Autodesk Fusion 360 part; units mm, degrees
(part 5 of 8)
  line L594 (-322.3503, 58.85) -> (-319.3503, 58.85)
  line L595 (-319.3503, 58.85) -> (-319.3503, 55.85)
  line L596 (-319.3503, 55.85) -> (-322.3503, 55.85)
  line L597 (-322.3503, 55.85) -> (-322.3503, 52.85)
  line L598 (-322.3503, 52.85) -> (-319.3503, 52.85)
  line L599 (-319.3503, 52.85) -> (-319.3503, 49.85)
  line L600 (-319.3503, 49.85) -> (-322.3503, 49.85)
  line L601 (-322.3503, 49.85) -> (-322.3503, 46.85)
  line L602 (-322.3503, 46.85) -> (-319.3503, 46.85)
  line L603 (-319.3503, 46.85) -> (-319.3503, 43.85)
  line L604 (-319.3503, 43.85) -> (-322.3503, 43.85)
  line L605 (-322.3503, 43.85) -> (-322.3503, 40.85)
  line L606 (-322.3503, 40.85) -> (-319.3503, 40.85)
  line L607 (-319.3503, 40.85) -> (-319.3503, 37.85)
  line L608 (-319.3503, 37.85) -> (-322.3503, 37.85)
  line L609 (-322.3503, 37.85) -> (-322.3503, 34.85)
  line L610 (-322.3503, 34.85) -> (-319.3503, 34.85)
  line L611 (-319.3503, 34.85) -> (-319.3503, 31.85)
  circle A0 centre (-110.4882, 52.6046) radius 2.5
  circle A1 centre (-197.9882, 140.1046) radius 2.5
  circle A2 centre (-210.4882, 152.6046) radius 2.5
  circle A3 centre (-122.9882, 65.1046) radius 2.5
  circle A4 centre (-122.9882, 140.1046) radius 2.5
  circle A5 centre (-197.9882, 65.1046) radius 2.5
  circle A6 centre (-210.4882, 52.6046) radius 2.5
  circle A7 centre (-110.4882, 152.6046) radius 2.5
sketch "Sketch8" plane through (0, 3, 0) normal (0, 1, 0) x (-1, 0, 0)
  line L0 (-319.3503, 31.85) -> (-322.3503, 31.85)
  line L1 (-322.3503, 31.85) -> (-322.3503, 28.1)
  line L2 (-322.3503, 28.1) -> (-319.3503, 28.1)
  line L3 (-319.3503, 28.1) -> (-319.3503, 27.35)
  line L4 (-319.3503, 27.35) -> (-317.6003, 27.35)
  line L5 (-317.6003, 27.35) -> (-317.6003, 24.35)
  line L6 (-317.6003, 24.35) -> (-312.8503, 24.35)
  line L7 (-312.8503, 24.35) -> (-312.8503, 27.35)
  line L8 (-312.8503, 27.35) -> (-309.8503, 27.35)
  line L9 (-309.8503, 27.35) -> (-309.8503, 24.35)
  line L10 (-309.8503, 24.35) -> (-306.8503, 24.35)
  line L11 (-306.8503, 24.35) -> (-306.8503, 27.35)
  line L12 (-306.8503, 27.35) -> (-303.8502, 27.35)
  line L13 (-303.8502, 27.35) -> (-303.8502, 24.35)
  line L14 (-303.8502, 24.35) -> (-300.8502, 24.35)
  line L15 (-300.8502, 24.35) -> (-300.8502, 27.35)
  line L16 (-300.8502, 27.35) -> (-297.8502, 27.35)
  line L17 (-297.8502, 27.35) -> (-297.8502, 24.35)
  line L18 (-297.8502, 24.35) -> (-294.8502, 24.35)
  line L19 (-294.8502, 24.35) -> (-294.8502, 27.35)
  line L20 (-294.8502, 27.35) -> (-291.8502, 27.35)
  line L21 (-291.8502, 27.35) -> (-291.8502, 24.35)
  line L22 (-291.8502, 24.35) -> (-288.8502, 24.35)
  line L23 (-288.8502, 24.35) -> (-288.8502, 27.35)
  line L24 (-288.8502, 27.35) -> (-285.8502, 27.35)
  line L25 (-285.8502, 27.35) -> (-285.8502, 24.35)
  line L26 (-285.8502, 24.35) -> (-282.8502, 24.35)
  line L27 (-282.8502, 24.35) -> (-282.8502, 27.35)
  line L28 (-282.8502, 27.35) -> (-279.8502, 27.35)
  line L29 (-279.8502, 27.35) -> (-279.8502, 24.35)
  line L30 (-279.8502, 24.35) -> (-276.8502, 24.35)
  line L31 (-276.8502, 24.35) -> (-276.8502, 27.35)
  line L32 (-276.8502, 27.35) -> (-273.8502, 27.35)
  line L33 (-273.8502, 27.35) -> (-273.8502, 24.35)
  line L34 (-273.8502, 24.35) -> (-270.8502, 24.35)
  line L35 (-270.8502, 24.35) -> (-270.8502, 27.35)
  line L36 (-270.8502, 27.35) -> (-267.8502, 27.35)
  line L37 (-267.8502, 27.35) -> (-267.8502, 24.35)
  line L38 (-267.8502, 24.35) -> (-264.8502, 24.35)
  line L39 (-264.8502, 24.35) -> (-264.8502, 27.35)
  line L40 (-264.8502, 27.35) -> (-261.8502, 27.35)
  line L41 (-261.8502, 27.35) -> (-261.8502, 24.35)
  line L42 (-261.8502, 24.35) -> (-258.8502, 24.35)
  line L43 (-258.8502, 24.35) -> (-258.8502, 27.35)
  line L44 (-258.8502, 27.35) -> (-255.8502, 27.35)
  line L45 (-255.8502, 27.35) -> (-255.8502, 24.35)
  line L46 (-255.8502, 24.35) -> (-252.8502, 24.35)
  line L47 (-252.8502, 24.35) -> (-252.8502, 27.35)
  line L48 (-252.8502, 27.35) -> (-249.8502, 27.35)
  line L49 (-249.8502, 27.35) -> (-249.8502, 24.35)
  line L50 (-249.8502, 24.35) -> (-246.8502, 24.35)
  line L51 (-246.8502, 24.35) -> (-246.8502, 27.35)
  line L52 (-246.8502, 27.35) -> (-243.8502, 27.35)
  line L53 (-243.8502, 27.35) -> (-243.8502, 24.35)
  line L54 (-243.8502, 24.35) -> (-240.8502, 24.35)
  line L55 (-240.8502, 24.35) -> (-240.8502, 27.35)
  line L56 (-240.8502, 27.35) -> (-237.8502, 27.35)
  line L57 (-237.8502, 27.35) -> (-237.8502, 24.35)
  line L58 (-237.8502, 24.35) -> (-234.8502, 24.35)
  line L59 (-234.8502, 24.35) -> (-234.8502, 27.35)
  line L60 (-234.8502, 27.35) -> (-231.8502, 27.35)
  line L61 (-231.8502, 27.35) -> (-231.8502, 24.35)
  line L62 (-231.8502, 24.35) -> (-228.8502, 24.35)
  line L63 (-228.8502, 24.35) -> (-228.8502, 27.35)
  line L64 (-228.8502, 27.35) -> (-225.8502, 27.35)
  line L65 (-225.8502, 27.35) -> (-225.8502, 24.35)
  line L66 (-225.8502, 24.35) -> (-222.8502, 24.35)
  line L67 (-222.8502, 24.35) -> (-222.8502, 27.35)
  line L68 (-222.8502, 27.35) -> (-219.8502, 27.35)
  line L69 (-219.8502, 27.35) -> (-219.8502, 24.35)
  line L70 (-219.8502, 24.35) -> (-216.8502, 24.35)
  line L71 (-216.8502, 24.35) -> (-216.8502, 27.35)
  line L72 (-216.8502, 27.35) -> (-213.8502, 27.35)
  line L73 (-213.8502, 27.35) -> (-213.8502, 24.35)
  line L74 (-213.8502, 24.35) -> (-210.8502, 24.35)
  line L75 (-210.8502, 24.35) -> (-210.8502, 27.35)
  line L76 (-210.8502, 27.35) -> (-207.8502, 27.35)
  line L77 (-207.8502, 27.35) -> (-207.8502, 24.35)
  line L78 (-207.8502, 24.35) -> (-204.8502, 24.35)
  line L79 (-204.8502, 24.35) -> (-204.8502, 27.35)
  line L80 (-204.8502, 27.35) -> (-201.8502, 27.35)
  line L81 (-201.8502, 27.35) -> (-201.8502, 24.35)
  line L82 (-201.8502, 24.35) -> (-198.8502, 24.35)
  line L83 (-198.8502, 24.35) -> (-198.8502, 27.35)
  line L84 (-198.8502, 27.35) -> (-195.8502, 27.35)
  line L85 (-195.8502, 27.35) -> (-195.8502, 24.35)
  line L86 (-195.8502, 24.35) -> (-192.8502, 24.35)
  line L87 (-192.8502, 24.35) -> (-192.8502, 27.35)
  line L88 (-192.8502, 27.35) -> (-189.8502, 27.35)
  line L89 (-189.8502, 27.35) -> (-189.8502, 24.35)
  line L90 (-189.8502, 24.35) -> (-186.8502, 24.35)
  line L91 (-186.8502, 24.35) -> (-186.8502, 27.35)
  line L92 (-186.8502, 27.35) -> (-183.8502, 27.35)
  line L93 (-183.8502, 27.35) -> (-183.8502, 24.35)
  line L94 (-183.8502, 24.35) -> (-180.8501, 24.35)
  line L95 (-180.8501, 24.35) -> (-180.8501, 27.35)
  line L96 (-180.8501, 27.35) -> (-177.8501, 27.35)
  line L97 (-177.8501, 27.35) -> (-177.8501, 24.35)
  line L98 (-177.8501, 24.35) -> (-174.8501, 24.35)
  line L99 (-174.8501, 24.35) -> (-174.8501, 27.35)
  line L100 (-174.8501, 27.35) -> (-171.8501, 27.35)
  line L101 (-171.8501, 27.35) -> (-171.8501, 24.35)
  line L102 (-171.8501, 24.35) -> (-168.8501, 24.35)
  line L103 (-168.8501, 24.35) -> (-168.8501, 27.35)
  line L104 (-168.8501, 27.35) -> (-165.8501, 27.35)
  line L105 (-165.8501, 27.35) -> (-165.8501, 24.35)
  line L106 (-165.8501, 24.35) -> (-162.8501, 24.35)
  line L107 (-162.8501, 24.35) -> (-162.8501, 27.35)
  line L108 (-162.8501, 27.35) -> (-159.8501, 27.35)
  line L109 (-159.8501, 27.35) -> (-159.8501, 24.35)
  line L110 (-159.8501, 24.35) -> (-156.8501, 24.35)
  line L111 (-156.8501, 24.35) -> (-156.8501, 27.35)
  line L112 (-156.8501, 27.35) -> (-153.8501, 27.35)
  line L113 (-153.8501, 27.35) -> (-153.8501, 24.35)
  line L114 (-153.8501, 24.35) -> (-150.8501, 24.35)
  line L115 (-150.8501, 24.35) -> (-150.8501, 27.35)
  line L116 (-150.8501, 27.35) -> (-147.8501, 27.35)
  line L117 (-147.8501, 27.35) -> (-147.8501, 24.35)
  line L118 (-147.8501, 24.35) -> (-144.8501, 24.35)
  line L119 (-144.8501, 24.35) -> (-144.8501, 27.35)
  line L120 (-144.8501, 27.35) -> (-141.8501, 27.35)
  line L121 (-141.8501, 27.35) -> (-141.8501, 24.35)
  line L122 (-141.8501, 24.35) -> (-138.8501, 24.35)
  line L123 (-138.8501, 24.35) -> (-138.8501, 27.35)
  line L124 (-138.8501, 27.35) -> (-135.8501, 27.35)
  line L125 (-135.8501, 27.35) -> (-135.8501, 24.35)
  line L126 (-135.8501, 24.35) -> (-132.8501, 24.35)
  line L127 (-132.8501, 24.35) -> (-132.8501, 27.35)
  line L128 (-132.8501, 27.35) -> (-129.8501, 27.35)
  line L129 (-129.8501, 27.35) -> (-129.8501, 24.35)
  line L130 (-129.8501, 24.35) -> (-126.8501, 24.35)
  line L131 (-126.8501, 24.35) -> (-126.8501, 27.35)
  line L132 (-126.8501, 27.35) -> (-123.8501, 27.35)
  line L133 (-123.8501, 27.35) -> (-123.8501, 24.35)
  line L134 (-123.8501, 24.35) -> (-120.8501, 24.35)
  line L135 (-120.8501, 24.35) -> (-120.8501, 27.35)
  line L136 (-120.8501, 27.35) -> (-117.8501, 27.35)
  line L137 (-117.8501, 27.35) -> (-117.8501, 24.35)
  line L138 (-117.8501, 24.35) -> (-114.8501, 24.35)
  line L139 (-114.8501, 24.35) -> (-114.8501, 27.35)
  line L140 (-114.8501, 27.35) -> (-111.8501, 27.35)
  line L141 (-111.8501, 27.35) -> (-111.8501, 24.35)
  line L142 (-111.8501, 24.35) -> (-108.8501, 24.35)
  line L143 (-108.8501, 24.35) -> (-108.8501, 27.35)
  line L144 (-108.8501, 27.35) -> (-105.8501, 27.35)
  line L145 (-105.8501, 27.35) -> (-105.8501, 24.35)
  line L146 (-105.8501, 24.35) -> (-102.8501, 24.35)
  line L147 (-102.8501, 24.35) -> (-102.8501, 27.35)
  line L148 (-102.8501, 27.35) -> (-99.8501, 27.35)
  line L149 (-99.8501, 27.35) -> (-99.8501, 24.35)
  line L150 (-99.8501, 24.35) -> (-96.8501, 24.35)
  line L151 (-96.8501, 24.35) -> (-96.8501, 27.35)
  line L152 (-96.8501, 27.35) -> (-93.8501, 27.35)
  line L153 (-93.8501, 27.35) -> (-93.8501, 24.35)
  line L154 (-93.8501, 24.35) -> (-90.8501, 24.35)
  line L155 (-90.8501, 24.35) -> (-90.8501, 27.35)
  line L156 (-90.8501, 27.35) -> (-87.8501, 27.35)
  line L157 (-87.8501, 27.35) -> (-87.8501, 24.35)
  line L158 (-87.8501, 24.35) -> (-84.8501, 24.35)
  line L159 (-84.8501, 24.35) -> (-84.8501, 27.35)
  line L160 (-84.8501, 27.35) -> (-81.8501, 27.35)
  line L161 (-81.8501, 27.35) -> (-81.8501, 24.35)
  line L162 (-81.8501, 24.35) -> (-78.8501, 24.35)
  line L163 (-78.8501, 24.35) -> (-78.8501, 27.35)
  line L164 (-78.8501, 27.35) -> (-75.8501, 27.35)
  line L165 (-75.8501, 27.35) -> (-75.8501, 24.35)
  line L166 (-75.8501, 24.35) -> (-72.8501, 24.35)
  line L167 (-72.8501, 24.35) -> (-72.8501, 27.35)
  line L168 (-72.8501, 27.35) -> (-69.8501, 27.35)
  line L169 (-69.8501, 27.35) -> (-69.8501, 24.35)
  line L170 (-69.8501, 24.35) -> (-66.8501, 24.35)
  line L171 (-66.8501, 24.35) -> (-66.8501, 27.35)
  line L172 (-66.8501, 27.35) -> (-63.8501, 27.35)
  line L173 (-63.8501, 27.35) -> (-63.8501, 24.35)
  line L174 (-63.8501, 24.35) -> (-60.8501, 24.35)
  line L175 (-60.8501, 24.35) -> (-60.8501, 27.35)
  line L176 (-60.8501, 27.35) -> (-57.85, 27.35)
  line L177 (-57.85, 27.35) -> (-57.85, 24.35)
  line L178 (-57.85, 24.35) -> (-54.85, 24.35)
  line L179 (-54.85, 24.35) -> (-54.85, 27.35)
  line L180 (-54.85, 27.35) -> (-51.85, 27.35)
  line L181 (-51.85, 27.35) -> (-51.85, 24.35)
  line L182 (-51.85, 24.35) -> (-48.85, 24.35)
  line L183 (-48.85, 24.35) -> (-48.85, 27.35)
  line L184 (-48.85, 27.35) -> (-45.85, 27.35)
  line L185 (-45.85, 27.35) -> (-45.85, 24.35)
  line L186 (-45.85, 24.35) -> (-42.85, 24.35)
  line L187 (-42.85, 24.35) -> (-42.85, 27.35)
  line L188 (-42.85, 27.35) -> (-39.85, 27.35)
  line L189 (-39.85, 27.35) -> (-39.85, 24.35)
  line L190 (-39.85, 24.35) -> (-36.85, 24.35)
  line L191 (-36.85, 24.35) -> (-36.85, 27.35)
  line L192 (-36.85, 27.35) -> (-33.85, 27.35)
  line L193 (-33.85, 27.35) -> (-33.85, 24.35)
  line L194 (-33.85, 24.35) -> (-30.85, 24.35)
  line L195 (-30.85, 24.35) -> (-30.85, 27.35)
  line L196 (-30.85, 27.35) -> (-27.85, 27.35)
  line L197 (-27.85, 27.35) -> (-27.85, 24.35)
  line L198 (-27.85, 24.35) -> (-24.85, 24.35)
  line L199 (-24.85, 24.35) -> (-24.85, 27.35)
  line L200 (-24.85, 27.35) -> (-21.85, 27.35)
  line L201 (-21.85, 27.35) -> (-21.85, 24.35)
  line L202 (-21.85, 24.35) -> (-18.85, 24.35)
  line L203 (-18.85, 24.35) -> (-18.85, 27.35)
  line L204 (-18.85, 27.35) -> (-15.85, 27.35)
  line L205 (-15.85, 27.35) -> (-15.85, 24.35)
  line L206 (-15.85, 24.35) -> (-11.1, 24.35)
  line L207 (-11.1, 24.35) -> (-11.1, 27.35)
  line L208 (-11.1, 27.35) -> (-9.35, 27.35)
  line L209 (-9.35, 27.35) -> (-9.35, 28.1)
  line L210 (-9.35, 28.1) -> (-6.35, 28.1)
  line L211 (-6.35, 28.1) -> (-6.35, 31.85)
  line L212 (-6.35, 31.85) -> (-9.35, 31.85)
  line L213 (-9.35, 31.85) -> (-9.35, 34.85)
  line L214 (-9.35, 34.85) -> (-6.35, 34.85)
  line L215 (-6.35, 34.85) -> (-6.35, 37.85)
  line L216 (-6.35, 37.85) -> (-9.35, 37.85)
  line L217 (-9.35, 37.85) -> (-9.35, 40.85)
  line L218 (-9.35, 40.85) -> (-6.35, 40.85)
  line L219 (-6.35, 40.85) -> (-6.35, 43.85)
  line L220 (-6.35, 43.85) -> (-9.35, 43.85)
  line L221 (-9.35, 43.85) -> (-9.35, 46.85)
  line L222 (-9.35, 46.85) -> (-6.35, 46.85)
  line L223 (-6.35, 46.85) -> (-6.35, 49.85)
  line L224 (-6.35, 49.85) -> (-9.35, 49.85)
  line L225 (-9.35, 49.85) -> (-9.35, 52.85)
  line L226 (-9.35, 52.85) -> (-6.35, 52.85)
  line L227 (-6.35, 52.85) -> (-6.35, 55.85)
  line L228 (-6.35, 55.85) -> (-9.35, 55.85)
  line L229 (-9.35, 55.85) -> (-9.35, 58.85)
  line L230 (-9.35, 58.85) -> (-6.35, 58.85)
  line L231 (-6.35, 58.85) -> (-6.35, 61.8501)
  line L232 (-6.35, 61.8501) -> (-9.35, 61.8501)
  line L233 (-9.35, 61.8501) -> (-9.35, 64.8501)
  line L234 (-9.35, 64.8501) -> (-6.35, 64.8501)
  line L235 (-6.35, 64.8501) -> (-6.35, 67.8501)
  line L236 (-6.35, 67.8501) -> (-9.35, 67.8501)
  line L237 (-9.35, 67.8501) -> (-9.35, 70.8501)
  line L238 (-9.35, 70.8501) -> (-6.35, 70.8501)
  line L239 (-6.35, 70.8501) -> (-6.35, 73.8501)
  line L240 (-6.35, 73.8501) -> (-9.35, 73.8501)
  line L241 (-9.35, 73.8501) -> (-9.35, 76.8501)
  line L242 (-9.35, 76.8501) -> (-6.35, 76.8501)
  line L243 (-6.35, 76.8501) -> (-6.35, 79.8501)
  line L244 (-6.35, 79.8501) -> (-9.35, 79.8501)
  line L245 (-9.35, 79.8501) -> (-9.35, 82.8501)
  line L246 (-9.35, 82.8501) -> (-6.35, 82.8501)
  line L247 (-6.35, 82.8501) -> (-6.35, 85.8501)
  line L248 (-6.35, 85.8501) -> (-9.35, 85.8501)
  line L249 (-9.35, 85.8501) -> (-9.35, 88.8501)
  line L250 (-9.35, 88.8501) -> (-6.35, 88.8501)
  line L251 (-6.35, 88.8501) -> (-6.35, 91.8501)
  line L252 (-6.35, 91.8501) -> (-9.35, 91.8501)
  line L253 (-9.35, 91.8501) -> (-9.35, 94.8501)
  line L254 (-9.35, 94.8501) -> (-6.35, 94.8501)
  line L255 (-6.35, 94.8501) -> (-6.35, 97.8501)
  line L256 (-6.35, 97.8501) -> (-9.35, 97.8501)
  line L257 (-9.35, 97.8501) -> (-9.35, 100.8501)
  line L258 (-9.35, 100.8501) -> (-6.35, 100.8501)
  line L259 (-6.35, 100.8501) -> (-6.35, 103.8501)
  line L260 (-6.35, 103.8501) -> (-9.35, 103.8501)
  line L261 (-9.35, 103.8501) -> (-9.35, 106.8501)
  line L262 (-9.35, 106.8501) -> (-6.35, 106.8501)
  line L263 (-6.35, 106.8501) -> (-6.35, 109.8501)
  line L264 (-6.35, 109.8501) -> (-9.35, 109.8501)
  line L265 (-9.35, 109.8501) -> (-9.35, 112.8501)
  line L266 (-9.35, 112.8501) -> (-6.35, 112.8501)
  line L267 (-6.35, 112.8501) -> (-6.35, 115.8501)
  line L268 (-6.35, 115.8501) -> (-9.35, 115.8501)
  line L269 (-9.35, 115.8501) -> (-9.35, 118.8501)
  line L270 (-9.35, 118.8501) -> (-6.35, 118.8501)
  line L271 (-6.35, 118.8501) -> (-6.35, 121.8501)
  line L272 (-6.35, 121.8501) -> (-9.35, 121.8501)
  line L273 (-9.35, 121.8501) -> (-9.35, 124.8501)
  line L274 (-9.35, 124.8501) -> (-6.35, 124.8501)
  line L275 (-6.35, 124.8501) -> (-6.35, 127.8501)
  line L276 (-6.35, 127.8501) -> (-9.35, 127.8501)
  line L277 (-9.35, 127.8501) -> (-9.35, 130.8501)
  line L278 (-9.35, 130.8501) -> (-6.35, 130.8501)
  line L279 (-6.35, 130.8501) -> (-6.35, 133.8501)
  line L280 (-6.35, 133.8501) -> (-9.35, 133.8501)
  line L281 (-9.35, 133.8501) -> (-9.35, 136.8501)
  line L282 (-9.35, 136.8501) -> (-6.35, 136.8501)
  line L283 (-6.35, 136.8501) -> (-6.35, 139.8501)
  line L284 (-6.35, 139.8501) -> (-9.35, 139.8501)
  line L285 (-9.35, 139.8501) -> (-9.35, 142.8501)
  line L286 (-9.35, 142.8501) -> (-6.35, 142.8501)
  line L287 (-6.35, 142.8501) -> (-6.35, 145.8501)
  line L288 (-6.35, 145.8501) -> (-9.35, 145.8501)
  line L289 (-9.35, 145.8501) -> (-9.35, 148.8501)
  line L290 (-9.35, 148.8501) -> (-6.35, 148.8501)
  line L291 (-6.35, 148.8501) -> (-6.35, 151.8501)
  line L292 (-6.35, 151.8501) -> (-9.35, 151.8501)
  line L293 (-9.35, 151.8501) -> (-9.35, 154.8501)
  line L294 (-9.35, 154.8501) -> (-6.35, 154.8501)
  line L295 (-6.35, 154.8501) -> (-6.35, 157.8501)
  line L296 (-6.35, 157.8501) -> (-9.35, 157.8501)
  line L297 (-9.35, 157.8501) -> (-9.35, 160.8501)
  line L298 (-9.35, 160.8501) -> (-6.35, 160.8501)
  line L299 (-6.35, 160.8501) -> (-6.35, 163.8501)
  line L300 (-6.35, 163.8501) -> (-9.35, 163.8501)
  line L301 (-9.35, 163.8501) -> (-9.35, 166.8501)
  line L302 (-9.35, 166.8501) -> (-6.35, 166.8501)
  line L303 (-6.35, 166.8501) -> (-6.35, 169.8501)
  line L304 (-6.35, 169.8501) -> (-9.35, 169.8501)
  line L305 (-9.35, 169.8501) -> (-9.35, 172.8501)
  line L306 (-9.35, 172.8501) -> (-6.35, 172.8501)
  line L307 (-6.35, 172.8501) -> (-6.35, 176.6001)
  line L308 (-6.35, 176.6001) -> (-9.35, 176.6001)
  line L309 (-9.35, 176.6001) -> (-9.35, 177.3501)
  line L310 (-9.35, 177.3501) -> (-11.1, 177.3501)
  line L311 (-11.1, 177.3501) -> (-11.1, 180.3501)
  line L312 (-11.1, 180.3501) -> (-15.85, 180.3501)
  line L313 (-15.85, 180.3501) -> (-15.85, 177.3501)
  line L314 (-15.85, 177.3501) -> (-18.85, 177.3501)
  line L315 (-18.85, 177.3501) -> (-18.85, 180.3501)
  line L316 (-18.85, 180.3501) -> (-21.85, 180.3501)
  line L317 (-21.85, 180.3501) -> (-21.85, 177.3501)
  line L318 (-21.85, 177.3501) -> (-24.85, 177.3501)
  line L319 (-24.85, 177.3501) -> (-24.85, 180.3501)
  line L320 (-24.85, 180.3501) -> (-27.85, 180.3501)
  line L321 (-27.85, 180.3501) -> (-27.85, 177.3501)
  line L322 (-27.85, 177.3501) -> (-30.85, 177.3501)
  line L323 (-30.85, 177.3501) -> (-30.85, 180.3501)
  line L324 (-30.85, 180.3501) -> (-33.85, 180.3501)
  line L325 (-33.85, 180.3501) -> (-33.85, 177.3501)
  line L326 (-33.85, 177.3501) -> (-36.85, 177.3501)
  line L327 (-36.85, 177.3501) -> (-36.85, 180.3501)
  line L328 (-36.85, 180.3501) -> (-39.85, 180.3501)
  line L329 (-39.85, 180.3501) -> (-39.85, 177.3501)
  line L330 (-39.85, 177.3501) -> (-42.85, 177.3501)
  line L331 (-42.85, 177.3501) -> (-42.85, 180.3501)
  line L332 (-42.85, 180.3501) -> (-45.85, 180.3501)
  line L333 (-45.85, 180.3501) -> (-45.85, 177.3501)
  line L334 (-45.85, 177.3501) -> (-48.85, 177.3501)
  line L335 (-48.85, 177.3501) -> (-48.85, 180.3501)
  line L336 (-48.85, 180.3501) -> (-51.85, 180.3501)
  line L337 (-51.85, 180.3501) -> (-51.85, 177.3501)
  line L338 (-51.85, 177.3501) -> (-54.85, 177.3501)
  line L339 (-54.85, 177.3501) -> (-54.85, 180.3501)
  line L340 (-54.85, 180.3501) -> (-57.85, 180.3501)
  line L341 (-57.85, 180.3501) -> (-57.85, 177.3501)
  line L342 (-57.85, 177.3501) -> (-60.8501, 177.3501)
  line L343 (-60.8501, 177.3501) -> (-60.8501, 180.3501)
  line L344 (-60.8501, 180.3501) -> (-63.8501, 180.3501)
  line L345 (-63.8501, 180.3501) -> (-63.8501, 177.3501)
  line L346 (-63.8501, 177.3501) -> (-66.8501, 177.3501)
  line L347 (-66.8501, 177.3501) -> (-66.8501, 180.3501)
  line L348 (-66.8501, 180.3501) -> (-69.8501, 180.3501)
  line L349 (-69.8501, 180.3501) -> (-69.8501, 177.3501)
  line L350 (-69.8501, 177.3501) -> (-72.8501, 177.3501)
  line L351 (-72.8501, 177.3501) -> (-72.8501, 180.3501)
  line L352 (-72.8501, 180.3501) -> (-75.8501, 180.3501)
  line L353 (-75.8501, 180.3501) -> (-75.8501, 177.3501)
  line L354 (-75.8501, 177.3501) -> (-78.8501, 177.3501)
  line L355 (-78.8501, 177.3501) -> (-78.8501, 180.3501)
  line L356 (-78.8501, 180.3501) -> (-81.8501, 180.3501)
  line L357 (-81.8501, 180.3501) -> (-81.8501, 177.3501)
  line L358 (-81.8501, 177.3501) -> (-84.8501, 177.3501)
  line L359 (-84.8501, 177.3501) -> (-84.8501, 180.3501)
  line L360 (-84.8501, 180.3501) -> (-87.8501, 180.3501)
  line L361 (-87.8501, 180.3501) -> (-87.8501, 177.3501)
  line L362 (-87.8501, 177.3501) -> (-90.8501, 177.3501)
  line L363 (-90.8501, 177.3501) -> (-90.8501, 180.3501)
  line L364 (-90.8501, 180.3501) -> (-93.8501, 180.3501)
  line L365 (-93.8501, 180.3501) -> (-93.8501, 177.3501)
  line L366 (-93.8501, 177.3501) -> (-96.8501, 177.3501)
  line L367 (-96.8501, 177.3501) -> (-96.8501, 180.3501)
  line L368 (-96.8501, 180.3501) -> (-99.8501, 180.3501)
  line L369 (-99.8501, 180.3501) -> (-99.8501, 177.3501)
  line L370 (-99.8501, 177.3501) -> (-102.8501, 177.3501)
  line L371 (-102.8501, 177.3501) -> (-102.8501, 180.3501)
  line L372 (-102.8501, 180.3501) -> (-105.8501, 180.3501)
  line L373 (-105.8501, 180.3501) -> (-105.8501, 177.3501)
  line L374 (-105.8501, 177.3501) -> (-108.8501, 177.3501)
  line L375 (-108.8501, 177.3501) -> (-108.8501, 180.3501)
  line L376 (-108.8501, 180.3501) -> (-111.8501, 180.3501)
  line L377 (-111.8501, 180.3501) -> (-111.8501, 177.3501)
  line L378 (-111.8501, 177.3501) -> (-114.8501, 177.3501)
  line L379 (-114.8501, 177.3501) -> (-114.8501, 180.3501)
  line L380 (-114.8501, 180.3501) -> (-117.8501, 180.3501)
  line L381 (-117.8501, 180.3501) -> (-117.8501, 177.3501)
  line L382 (-117.8501, 177.3501) -> (-120.8501, 177.3501)
  line L383 (-120.8501, 177.3501) -> (-120.8501, 180.3501)
  line L384 (-120.8501, 180.3501) -> (-123.8501, 180.3501)
  line L385 (-123.8501, 180.3501) -> (-123.8501, 177.3501)
  line L386 (-123.8501, 177.3501) -> (-126.8501, 177.3501)
  line L387 (-126.8501, 177.3501) -> (-126.8501, 180.3501)
  line L388 (-126.8501, 180.3501) -> (-129.8501, 180.3501)
  line L389 (-129.8501, 180.3501) -> (-129.8501, 177.3501)
  line L390 (-129.8501, 177.3501) -> (-132.8501, 177.3501)
  line L391 (-132.8501, 177.3501) -> (-132.8501, 180.3501)
  line L392 (-132.8501, 180.3501) -> (-135.8501, 180.3501)
  line L393 (-135.8501, 180.3501) -> (-135.8501, 177.3501)
  line L394 (-135.8501, 177.3501) -> (-138.8501, 177.3501)
  line L395 (-138.8501, 177.3501) -> (-138.8501, 180.3501)
  line L396 (-138.8501, 180.3501) -> (-141.8501, 180.3501)
  line L397 (-141.8501, 180.3501) -> (-141.8501, 177.3501)
  line L398 (-141.8501, 177.3501) -> (-144.8501, 177.3501)
  line L399 (-144.8501, 177.3501) -> (-144.8501, 180.3501)
  line L400 (-144.8501, 180.3501) -> (-147.8501, 180.3501)
  line L401 (-147.8501, 180.3501) -> (-147.8501, 177.3501)
  line L402 (-147.8501, 177.3501) -> (-150.8501, 177.3501)
  line L403 (-150.8501, 177.3501) -> (-150.8501, 180.3501)
  line L404 (-150.8501, 180.3501) -> (-153.8501, 180.3501)
  line L405 (-153.8501, 180.3501) -> (-153.8501, 177.3501)
  line L406 (-153.8501, 177.3501) -> (-156.8501, 177.3501)
  line L407 (-156.8501, 177.3501) -> (-156.8501, 180.3501)
  line L408 (-156.8501, 180.3501) -> (-159.8501, 180.3501)
  line L409 (-159.8501, 180.3501) -> (-159.8501, 177.3501)
  line L410 (-159.8501, 177.3501) -> (-162.8501, 177.3501)
  line L411 (-162.8501, 177.3501) -> (-162.8501, 180.3501)
  line L412 (-162.8501, 180.3501) -> (-165.8501, 180.3501)
  line L413 (-165.8501, 180.3501) -> (-165.8501, 177.3501)
  line L414 (-165.8501, 177.3501) -> (-168.8501, 177.3501)
  line L415 (-168.8501, 177.3501) -> (-168.8501, 180.3501)
  line L416 (-168.8501, 180.3501) -> (-171.8501, 180.3501)
  line L417 (-171.8501, 180.3501) -> (-171.8501, 177.3501)
  line L418 (-171.8501, 177.3501) -> (-174.8501, 177.3501)
  line L419 (-174.8501, 177.3501) -> (-174.8501, 180.3501)
  line L420 (-174.8501, 180.3501) -> (-177.8501, 180.3501)
  line L421 (-177.8501, 180.3501) -> (-177.8501, 177.3501)
  line L422 (-177.8501, 177.3501) -> (-180.8501, 177.3501)
  line L423 (-180.8501, 177.3501) -> (-180.8501, 180.3501)
  line L424 (-180.8501, 180.3501) -> (-183.8502, 180.3501)
  line L425 (-183.8502, 180.3501) -> (-183.8502, 177.3501)
  line L426 (-183.8502, 177.3501) -> (-186.8502, 177.3501)
  line L427 (-186.8502, 177.3501) -> (-186.8502, 180.3501)
  line L428 (-186.8502, 180.3501) -> (-189.8502, 180.3501)
  line L429 (-189.8502, 180.3501) -> (-189.8502, 177.3501)
  line L430 (-189.8502, 177.3501) -> (-192.8502, 177.3501)
  line L431 (-192.8502, 177.3501) -> (-192.8502, 180.3501)
  line L432 (-192.8502, 180.3501) -> (-195.8502, 180.3501)
  line L433 (-195.8502, 180.3501) -> (-195.8502, 177.3501)
  line L434 (-195.8502, 177.3501) -> (-198.8502, 177.3501)
  line L435 (-198.8502, 177.3501) -> (-198.8502, 180.3501)
  line L436 (-198.8502, 180.3501) -> (-201.8502, 180.3501)
  line L437 (-201.8502, 180.3501) -> (-201.8502, 177.3501)
  line L438 (-201.8502, 177.3501) -> (-204.8502, 177.3501)
  line L439 (-204.8502, 177.3501) -> (-204.8502, 180.3501)
  line L440 (-204.8502, 180.3501) -> (-207.8502, 180.3501)
  line L441 (-207.8502, 180.3501) -> (-207.8502, 177.3501)
  line L442 (-207.8502, 177.3501) -> (-210.8502, 177.3501)
  line L443 (-210.8502, 177.3501) -> (-210.8502, 180.3501)
  line L444 (-210.8502, 180.3501) -> (-213.8502, 180.3501)
  line L445 (-213.8502, 180.3501) -> (-213.8502, 177.3501)
  line L446 (-213.8502, 177.3501) -> (-216.8502, 177.3501)
  line L447 (-216.8502, 177.3501) -> (-216.8502, 180.3501)
  line L448 (-216.8502, 180.3501) -> (-219.8502, 180.3501)
  line L449 (-219.8502, 180.3501) -> (-219.8502, 177.3501)
  line L450 (-219.8502, 177.3501) -> (-222.8502, 177.3501)
  line L451 (-222.8502, 177.3501) -> (-222.8502, 180.3501)
  line L452 (-222.8502, 180.3501) -> (-225.8502, 180.3501)
  line L453 (-225.8502, 180.3501) -> (-225.8502, 177.3501)
  line L454 (-225.8502, 177.3501) -> (-228.8502, 177.3501)
  line L455 (-228.8502, 177.3501) -> (-228.8502, 180.3501)
  line L456 (-228.8502, 180.3501) -> (-231.8502, 180.3501)
  line L457 (-231.8502, 180.3501) -> (-231.8502, 177.3501)
  line L458 (-231.8502, 177.3501) -> (-234.8502, 177.3501)
  line L459 (-234.8502, 177.3501) -> (-234.8502, 180.3501)
  line L460 (-234.8502, 180.3501) -> (-237.8502, 180.3501)
  line L461 (-237.8502, 180.3501) -> (-237.8502, 177.3501)
  line L462 (-237.8502, 177.3501) -> (-240.8502, 177.3501)
  line L463 (-240.8502, 177.3501) -> (-240.8502, 180.3501)
  line L464 (-240.8502, 180.3501) -> (-243.8502, 180.3501)
  line L465 (-243.8502, 180.3501) -> (-243.8502, 177.3501)
  line L466 (-243.8502, 177.3501) -> (-246.8502, 177.3501)
  line L467 (-246.8502, 177.3501) -> (-246.8502, 180.3501)
  line L468 (-246.8502, 180.3501) -> (-249.8502, 180.3501)
  line L469 (-249.8502, 180.3501) -> (-249.8502, 177.3501)
  line L470 (-249.8502, 177.3501) -> (-252.8502, 177.3501)
  line L471 (-252.8502, 177.3501) -> (-252.8502, 180.3501)
  line L472 (-252.8502, 180.3501) -> (-255.8502, 180.3501)
  line L473 (-255.8502, 180.3501) -> (-255.8502, 177.3501)
  line L474 (-255.8502, 177.3501) -> (-258.8502, 177.3501)
  line L475 (-258.8502, 177.3501) -> (-258.8502, 180.3501)
  line L476 (-258.8502, 180.3501) -> (-261.8502, 180.3501)
  line L477 (-261.8502, 180.3501) -> (-261.8502, 177.3501)
  line L478 (-261.8502, 177.3501) -> (-264.8502, 177.3501)
  line L479 (-264.8502, 177.3501) -> (-264.8502, 180.3501)
  line L480 (-264.8502, 180.3501) -> (-267.8502, 180.3501)
  line L481 (-267.8502, 180.3501) -> (-267.8502, 177.3501)
  line L482 (-267.8502, 177.3501) -> (-270.8502, 177.3501)
  line L483 (-270.8502, 177.3501) -> (-270.8502, 180.3501)
  line L484 (-270.8502, 180.3501) -> (-273.8502, 180.3501)
  line L485 (-273.8502, 180.3501) -> (-273.8502, 177.3501)
  line L486 (-273.8502, 177.3501) -> (-276.8502, 177.3501)
  line L487 (-276.8502, 177.3501) -> (-276.8502, 180.3501)
  line L488 (-276.8502, 180.3501) -> (-279.8502, 180.3501)
  line L489 (-279.8502, 180.3501) -> (-279.8502, 177.3501)
  line L490 (-279.8502, 177.3501) -> (-282.8502, 177.3501)
  line L491 (-282.8502, 177.3501) -> (-282.8502, 180.3501)
  line L492 (-282.8502, 180.3501) -> (-285.8502, 180.3501)
  line L493 (-285.8502, 180.3501) -> (-285.8502, 177.3501)
  line L494 (-285.8502, 177.3501) -> (-288.8502, 177.3501)
  line L495 (-288.8502, 177.3501) -> (-288.8502, 180.3501)
  line L496 (-288.8502, 180.3501) -> (-291.8502, 180.3501)
  line L497 (-291.8502, 180.3501) -> (-291.8502, 177.3501)
  line L498 (-291.8502, 177.3501) -> (-294.8502, 177.3501)
  line L499 (-294.8502, 177.3501) -> (-294.8502, 180.3501)
  line L500 (-294.8502, 180.3501) -> (-297.8502, 180.3501)
  line L501 (-297.8502, 180.3501) -> (-297.8502, 177.3501)
  line L502 (-297.8502, 177.3501) -> (-300.8502, 177.3501)
  line L503 (-300.8502, 177.3501) -> (-300.8502, 180.3501)
  line L504 (-300.8502, 180.3501) -> (-303.8502, 180.3501)
  line L505 (-303.8502, 180.3501) -> (-303.8502, 177.3501)
  line L506 (-303.8502, 177.3501) -> (-306.8503, 177.3501)
  line L507 (-306.8503, 177.3501) -> (-306.8503, 180.3501)
  line L508 (-306.8503, 180.3501) -> (-309.8503, 180.3501)
  line L509 (-309.8503, 180.3501) -> (-309.8503, 177.3501)
  line L510 (-309.8503, 177.3501) -> (-312.8503, 177.3501)
  line L511 (-312.8503, 177.3501) -> (-312.8503, 180.3501)
  line L512 (-312.8503, 180.3501) -> (-317.6003, 180.3501)
  line L513 (-317.6003, 180.3501) -> (-317.6003, 177.3501)
  line L514 (-317.6003, 177.3501) -> (-319.3503, 177.3501)
  line L515 (-319.3503, 177.3501) -> (-319.3503, 176.6001)
  line L516 (-319.3503, 176.6001) -> (-322.3503, 176.6001)
  line L517 (-322.3503, 176.6001) -> (-322.3503, 172.8501)
  line L518 (-322.3503, 172.8501) -> (-319.3503, 172.8501)
  line L519 (-319.3503, 172.8501) -> (-319.3503, 169.8501)
  line L520 (-319.3503, 169.8501) -> (-322.3503, 169.8501)
  line L521 (-322.3503, 169.8501) -> (-322.3503, 166.8501)
  line L522 (-322.3503, 166.8501) -> (-319.3503, 166.8501)
  line L523 (-319.3503, 166.8501) -> (-319.3503, 163.8501)
  line L524 (-319.3503, 163.8501) -> (-322.3503, 163.8501)
  line L525 (-322.3503, 163.8501) -> (-322.3503, 160.8501)
  line L526 (-322.3503, 160.8501) -> (-319.3503, 160.8501)
  line L527 (-319.3503, 160.8501) -> (-319.3503, 157.8501)
  line L528 (-319.3503, 157.8501) -> (-322.3503, 157.8501)
  line L529 (-322.3503, 157.8501) -> (-322.3503, 154.8501)
  line L530 (-322.3503, 154.8501) -> (-319.3503, 154.8501)
  line L531 (-319.3503, 154.8501) -> (-319.3503, 151.8501)
  line L532 (-319.3503, 151.8501) -> (-322.3503, 151.8501)
  line L533 (-322.3503, 151.8501) -> (-322.3503, 148.8501)
  line L534 (-322.3503, 148.8501) -> (-319.3503, 148.8501)
  line L535 (-319.3503, 148.8501) -> (-319.3503, 145.8501)
  line L536 (-319.3503, 145.8501) -> (-322.3503, 145.8501)
  line L537 (-322.3503, 145.8501) -> (-322.3503, 142.8501)
  line L538 (-322.3503, 142.8501) -> (-319.3503, 142.8501)
  line L539 (-319.3503, 142.8501) -> (-319.3503, 139.8501)
  line L540 (-319.3503, 139.8501) -> (-322.3503, 139.8501)
  line L541 (-322.3503, 139.8501) -> (-322.3503, 136.8501)
  line L542 (-322.3503, 136.8501) -> (-319.3503, 136.8501)
  line L543 (-319.3503, 136.8501) -> (-319.3503, 133.8501)
  line L544 (-319.3503, 133.8501) -> (-322.3503, 133.8501)
  line L545 (-322.3503, 133.8501) -> (-322.3503, 130.8501)
  line L546 (-322.3503, 130.8501) -> (-319.3503, 130.8501)
  line L547 (-319.3503, 130.8501) -> (-319.3503, 127.8501)
  line L548 (-319.3503, 127.8501) -> (-322.3503, 127.8501)
  line L549 (-322.3503, 127.8501) -> (-322.3503, 124.8501)
  line L550 (-322.3503, 124.8501) -> (-319.3503, 124.8501)
  line L551 (-319.3503, 124.8501) -> (-319.3503, 121.8501)
  line L552 (-319.3503, 121.8501) -> (-322.3503, 121.8501)
  line L553 (-322.3503, 121.8501) -> (-322.3503, 118.8501)
  line L554 (-322.3503, 118.8501) -> (-319.3503, 118.8501)
  line L555 (-319.3503, 118.8501) -> (-319.3503, 115.8501)
  line L556 (-319.3503, 115.8501) -> (-322.3503, 115.8501)
  line L557 (-322.3503, 115.8501) -> (-322.3503, 112.8501)
  line L558 (-322.3503, 112.8501) -> (-319.3503, 112.8501)
  line L559 (-319.3503, 112.8501) -> (-319.3503, 109.8501)
  line L560 (-319.3503, 109.8501) -> (-322.3503, 109.8501)
  line L561 (-322.3503, 109.8501) -> (-322.3503, 106.8501)
  line L562 (-322.3503, 106.8501) -> (-319.3503, 106.8501)
  line L563 (-319.3503, 106.8501) -> (-319.3503, 103.8501)
  line L564 (-319.3503, 103.8501) -> (-322.3503, 103.8501)
  line L565 (-322.3503, 103.8501) -> (-322.3503, 100.8501)
  line L566 (-322.3503, 100.8501) -> (-319.3503, 100.8501)
  line L567 (-319.3503, 100.8501) -> (-319.3503, 97.8501)
  line L568 (-319.3503, 97.8501) -> (-322.3503, 97.8501)
  line L569 (-322.3503, 97.8501) -> (-322.3503, 94.8501)
  line L570 (-322.3503, 94.8501) -> (-319.3503, 94.8501)
  line L571 (-319.3503, 94.8501) -> (-319.3503, 91.8501)
  line L572 (-319.3503, 91.8501) -> (-322.3503, 91.8501)
  line L573 (-322.3503, 91.8501) -> (-322.3503, 88.8501)
  line L574 (-322.3503, 88.8501) -> (-319.3503, 88.8501)
  line L575 (-319.3503, 88.8501) -> (-319.3503, 85.8501)
  line L576 (-319.3503, 85.8501) -> (-322.3503, 85.8501)
  line L577 (-322.3503, 85.8501) -> (-322.3503, 82.8501)
  line L578 (-322.3503, 82.8501) -> (-319.3503, 82.8501)
  line L579 (-319.3503, 82.8501) -> (-319.3503, 79.8501)
  line L580 (-319.3503, 79.8501) -> (-322.3503, 79.8501)
  line L581 (-322.3503, 79.8501) -> (-322.3503, 76.8501)
  line L582 (-322.3503, 76.8501) -> (-319.3503, 76.8501)
  line L583 (-319.3503, 76.8501) -> (-319.3503, 73.8501)
  line L584 (-319.3503, 73.8501) -> (-322.3503, 73.8501)
  line L585 (-322.3503, 73.8501) -> (-322.3503, 70.8501)
  line L586 (-322.3503, 70.8501) -> (-319.3503, 70.8501)
  line L587 (-319.3503, 70.8501) -> (-319.3503, 67.8501)
  line L588 (-319.3503, 67.8501) -> (-322.3503, 67.8501)
  line L589 (-322.3503, 67.8501) -> (-322.3503, 64.8501)
  line L590 (-322.3503, 64.8501) -> (-319.3503, 64.8501)
  line L591 (-319.3503, 64.8501) -> (-319.3503, 61.8501)
  line L592 (-319.3503, 61.8501) -> (-322.3503, 61.8501)
  line L593 (-322.3503, 61.8501) -> (-322.3503, 58.85)
  line L594 (-322.3503, 58.85) -> (-319.3503, 58.85)
  line L595 (-319.3503, 58.85) -> (-319.3503, 55.85)
  line L596 (-319.3503, 55.85) -> (-322.3503, 55.85)
  line L597 (-322.3503, 55.85) -> (-322.3503, 52.85)
  line L598 (-322.3503, 52.85) -> (-319.3503, 52.85)
  line L599 (-319.3503, 52.85) -> (-319.3503, 49.85)
  line L600 (-319.3503, 49.85) -> (-322.3503, 49.85)
  line L601 (-322.3503, 49.85) -> (-322.3503, 46.85)
  line L602 (-322.3503, 46.85) -> (-319.3503, 46.85)
  line L603 (-319.3503, 46.85) -> (-319.3503, 43.85)
  line L604 (-319.3503, 43.85) -> (-322.3503, 43.85)
  line L605 (-322.3503, 43.85) -> (-322.3503, 40.85)
  line L606 (-322.3503, 40.85) -> (-319.3503, 40.85)
  line L607 (-319.3503, 40.85) -> (-319.3503, 37.85)
  line L608 (-319.3503, 37.85) -> (-322.3503, 37.85)
  line L609 (-322.3503, 37.85) -> (-322.3503, 34.85)
  line L610 (-322.3503, 34.85) -> (-319.3503, 34.85)
  line L611 (-319.3503, 34.85) -> (-319.3503, 31.85)
  line L612 (-322.3503, 31.85, -3) -> (-319.3503, 31.85, -3)
  line L613 (-319.3503, 31.85, -3) -> (-319.3503, 34.85, -3)
  line L614 (-319.3503, 34.85, -3) -> (-322.3503, 34.85, -3)
  line L615 (-322.3503, 34.85, -3) -> (-322.3503, 37.85, -3)
  line L616 (-322.3503, 37.85, -3) -> (-319.3503, 37.85, -3)
  line L617 (-319.3503, 37.85, -3) -> (-319.3503, 40.85, -3)
  line L618 (-319.3503, 40.85, -3) -> (-322.3503, 40.85, -3)
  line L619 (-322.3503, 40.85, -3) -> (-322.3503, 43.85, -3)
  line L620 (-322.3503, 43.85, -3) -> (-319.3503, 43.85, -3)
  line L621 (-319.3503, 43.85, -3) -> (-319.3503, 46.85, -3)
  line L622 (-319.3503, 46.85, -3) -> (-322.3503, 46.85, -3)
  line L623 (-322.3503, 46.85, -3) -> (-322.3503, 49.85, -3)
  line L624 (-322.3503, 49.85, -3) -> (-319.3503, 49.85, -3)
  line L625 (-319.3503, 49.85, -3) -> (-319.3503, 52.85, -3)
  line L626 (-319.3503, 52.85, -3) -> (-322.3503, 52.85, -3)
  line L627 (-322.3503, 52.85, -3) -> (-322.3503, 55.85, -3)
  line L628 (-322.3503, 55.85, -3) -> (-319.3503, 55.85, -3)
  line L629 (-319.3503, 55.85, -3) -> (-319.3503, 58.85, -3)
  line L630 (-319.3503, 58.85, -3) -> (-322.3503, 58.85, -3)
  line L631 (-322.3503, 58.85, -3) -> (-322.3503, 61.8501, -3)
  line L632 (-322.3503, 61.8501, -3) -> (-319.3503, 61.8501, -3)
  line L633 (-319.3503, 61.8501, -3) -> (-319.3503, 64.8501, -3)
  line L634 (-319.3503, 64.8501, -3) -> (-322.3503, 64.8501, -3)
  line L635 (-322.3503, 64.8501, -3) -> (-322.3503, 67.8501, -3)
  line L636 (-322.3503, 67.8501, -3) -> (-319.3503, 67.8501, -3)
  line L637 (-319.3503, 67.8501, -3) -> (-319.3503, 70.8501, -3)
  line L638 (-319.3503, 70.8501, -3) -> (-322.3503, 70.8501, -3)
  line L639 (-322.3503, 70.8501, -3) -> (-322.3503, 73.8501, -3)
  line L640 (-322.3503, 73.8501, -3) -> (-319.3503, 73.8501, -3)
  line L641 (-319.3503, 73.8501, -3) -> (-319.3503, 76.8501, -3)
  line L642 (-319.3503, 76.8501, -3) -> (-322.3503, 76.8501, -3)
  line L643 (-322.3503, 76.8501, -3) -> (-322.3503, 79.8501, -3)
  line L644 (-322.3503, 79.8501, -3) -> (-319.3503, 79.8501, -3)
  line L645 (-319.3503, 79.8501, -3) -> (-319.3503, 82.8501, -3)
  line L646 (-319.3503, 82.8501, -3) -> (-322.3503, 82.8501, -3)
  line L647 (-322.3503, 82.8501, -3) -> (-322.3503, 85.8501, -3)
  line L648 (-322.3503, 85.8501, -3) -> (-319.3503, 85.8501, -3)
  line L649 (-319.3503, 85.8501, -3) -> (-319.3503, 88.8501, -3)
  line L650 (-319.3503, 88.8501, -3) -> (-322.3503, 88.8501, -3)
  line L651 (-322.3503, 88.8501, -3) -> (-322.3503, 91.8501, -3)
  line L652 (-322.3503, 91.8501, -3) -> (-319.3503, 91.8501, -3)
  line L653 (-319.3503, 91.8501, -3) -> (-319.3503, 94.8501, -3)
  line L654 (-319.3503, 94.8501, -3) -> (-322.3503, 94.8501, -3)
  line L655 (-322.3503, 94.8501, -3) -> (-322.3503, 97.8501, -3)
  line L656 (-322.3503, 97.8501, -3) -> (-319.3503, 97.8501, -3)
  line L657 (-319.3503, 97.8501, -3) -> (-319.3503, 100.8501, -3)
  line L658 (-319.3503, 100.8501, -3) -> (-322.3503, 100.8501, -3)
  line L659 (-322.3503, 100.8501, -3) -> (-322.3503, 103.8501, -3)
  line L660 (-322.3503, 103.8501, -3) -> (-319.3503, 103.8501, -3)
  line L661 (-319.3503, 103.8501, -3) -> (-319.3503, 106.8501, -3)
  line L662 (-319.3503, 106.8501, -3) -> (-322.3503, 106.8501, -3)
  line L663 (-322.3503, 106.8501, -3) -> (-322.3503, 109.8501, -3)
  line L664 (-322.3503, 109.8501, -3) -> (-319.3503, 109.8501, -3)
  line L665 (-319.3503, 109.8501, -3) -> (-319.3503, 112.8501, -3)
  line L666 (-319.3503, 112.8501, -3) -> (-322.3503, 112.8501, -3)
  line L667 (-322.3503, 112.8501, -3) -> (-322.3503, 115.8501, -3)
  line L668 (-322.3503, 115.8501, -3) -> (-319.3503, 115.8501, -3)
  line L669 (-319.3503, 115.8501, -3) -> (-319.3503, 118.8501, -3)
  line L670 (-319.3503, 118.8501, -3) -> (-322.3503, 118.8501, -3)
  line L671 (-322.3503, 118.8501, -3) -> (-322.3503, 121.8501, -3)
  line L672 (-322.3503, 121.8501, -3) -> (-319.3503, 121.8501, -3)
  line L673 (-319.3503, 121.8501, -3) -> (-319.3503, 124.8501, -3)
  line L674 (-319.3503, 124.8501, -3) -> (-322.3503, 124.8501, -3)
  line L675 (-322.3503, 124.8501, -3) -> (-322.3503, 127.8501, -3)
  line L676 (-322.3503, 127.8501, -3) -> (-319.3503, 127.8501, -3)
  line L677 (-319.3503, 127.8501, -3) -> (-319.3503, 130.8501, -3)
  line L678 (-319.3503, 130.8501, -3) -> (-322.3503, 130.8501, -3)
  line L679 (-322.3503, 130.8501, -3) -> (-322.3503, 133.8501, -3)
  line L680 (-322.3503, 133.8501, -3) -> (-319.3503, 133.8501, -3)
  line L681 (-319.3503, 133.8501, -3) -> (-319.3503, 136.8501, -3)
  line L682 (-319.3503, 136.8501, -3) -> (-322.3503, 136.8501, -3)
  line L683 (-322.3503, 136.8501, -3) -> (-322.3503, 139.8501, -3)
  line L684 (-322.3503, 139.8501, -3) -> (-319.3503, 139.8501, -3)
  line L685 (-319.3503, 139.8501, -3) -> (-319.3503, 142.8501, -3)
  line L686 (-319.3503, 142.8501, -3) -> (-322.3503, 142.8501, -3)
  line L687 (-322.3503, 142.8501, -3) -> (-322.3503, 145.8501, -3)
  line L688 (-322.3503, 145.8501, -3) -> (-319.3503, 145.8501, -3)
  line L689 (-319.3503, 145.8501, -3) -> (-319.3503, 148.8501, -3)
  line L690 (-319.3503, 148.8501, -3) -> (-322.3503, 148.8501, -3)
  line L691 (-322.3503, 148.8501, -3) -> (-322.3503, 151.8501, -3)
  line L692 (-322.3503, 151.8501, -3) -> (-319.3503, 151.8501, -3)
  line L693 (-319.3503, 151.8501, -3) -> (-319.3503, 154.8501, -3)
  line L694 (-319.3503, 154.8501, -3) -> (-322.3503, 154.8501, -3)
  line L695 (-322.3503, 154.8501, -3) -> (-322.3503, 157.8501, -3)
  line L696 (-322.3503, 157.8501, -3) -> (-319.3503, 157.8501, -3)
  line L697 (-319.3503, 157.8501, -3) -> (-319.3503, 160.8501, -3)
  line L698 (-319.3503, 160.8501, -3) -> (-322.3503, 160.8501, -3)
  line L699 (-322.3503, 160.8501, -3) -> (-322.3503, 163.8501, -3)
  line L700 (-322.3503, 163.8501, -3) -> (-319.3503, 163.8501, -3)
  line L701 (-319.3503, 163.8501, -3) -> (-319.3503, 166.8501, -3)
  line L702 (-319.3503, 166.8501, -3) -> (-322.3503, 166.8501, -3)
  line L703 (-322.3503, 166.8501, -3) -> (-322.3503, 169.8501, -3)
  line L704 (-322.3503, 169.8501, -3) -> (-319.3503, 169.8501, -3)
  line L705 (-319.3503, 169.8501, -3) -> (-319.3503, 172.8501, -3)
  line L706 (-319.3503, 172.8501, -3) -> (-322.3503, 172.8501, -3)
  line L707 (-322.3503, 172.8501, -3) -> (-322.3503, 176.6001, -3)
  line L708 (-322.3503, 176.6001, -3) -> (-319.3503, 176.6001, -3)
  line L709 (-319.3503, 176.6001, -3) -> (-319.3503, 177.3501, -3)
  line L710 (-319.3503, 177.3501, -3) -> (-317.6003, 177.3501, -3)
  line L711 (-317.6003, 177.3501, -3) -> (-317.6003, 180.3501, -3)
  line L712 (-317.6003, 180.3501, -3) -> (-312.8503, 180.3501, -3)
  line L713 (-312.8503, 180.3501, -3) -> (-312.8503, 177.3501, -3)
  line L714 (-312.8503, 177.3501, -3) -> (-309.8503, 177.3501, -3)
  line L715 (-309.8503, 177.3501, -3) -> (-309.8503, 180.3501, -3)
  line L716 (-309.8503, 180.3501, -3) -> (-306.8503, 180.3501, -3)
  line L717 (-306.8503, 180.3501, -3) -> (-306.8503, 177.3501, -3)
  line L718 (-306.8503, 177.3501, -3) -> (-303.8502, 177.3501, -3)
  line L719 (-303.8502, 177.3501, -3) -> (-303.8502, 180.3501, -3)
  line L720 (-303.8502, 180.3501, -3) -> (-300.8502, 180.3501, -3)
  line L721 (-300.8502, 180.3501, -3) -> (-300.8502, 177.3501, -3)
  line L722 (-300.8502, 177.3501, -3) -> (-297.8502, 177.3501, -3)
  line L723 (-297.8502, 177.3501, -3) -> (-297.8502, 180.3501, -3)
  line L724 (-297.8502, 180.3501, -3) -> (-294.8502, 180.3501, -3)
  line L725 (-294.8502, 180.3501, -3) -> (-294.8502, 177.3501, -3)
  line L726 (-294.8502, 177.3501, -3) -> (-291.8502, 177.3501, -3)
  line L727 (-291.8502, 177.3501, -3) -> (-291.8502, 180.3501, -3)
  line L728 (-291.8502, 180.3501, -3) -> (-288.8502, 180.3501, -3)
  line L729 (-288.8502, 180.3501, -3) -> (-288.8502, 177.3501, -3)
  line L730 (-288.8502, 177.3501, -3) -> (-285.8502, 177.3501, -3)
  line L731 (-285.8502, 177.3501, -3) -> (-285.8502, 180.3501, -3)
  line L732 (-285.8502, 180.3501, -3) -> (-282.8502, 180.3501, -3)
  line L733 (-282.8502, 180.3501, -3) -> (-282.8502, 177.3501, -3)
  line L734 (-282.8502, 177.3501, -3) -> (-279.8502, 177.3501, -3)
  line L735 (-279.8502, 177.3501, -3) -> (-279.8502, 180.3501, -3)
  line L736 (-279.8502, 180.3501, -3) -> (-276.8502, 180.3501, -3)
  line L737 (-276.8502, 180.3501, -3) -> (-276.8502, 177.3501, -3)
  line L738 (-276.8502, 177.3501, -3) -> (-273.8502, 177.3501, -3)
  line L739 (-273.8502, 177.3501, -3) -> (-273.8502, 180.3501, -3)
  line L740 (-273.8502, 180.3501, -3) -> (-270.8502, 180.3501, -3)
  line L741 (-270.8502, 180.3501, -3) -> (-270.8502, 177.3501, -3)
  line L742 (-270.8502, 177.3501, -3) -> (-267.8502, 177.3501, -3)
  line L743 (-267.8502, 177.3501, -3) -> (-267.8502, 180.3501, -3)
  line L744 (-267.8502, 180.3501, -3) -> (-264.8502, 180.3501, -3)
  line L745 (-264.8502, 180.3501, -3) -> (-264.8502, 177.3501, -3)
  line L746 (-264.8502, 177.3501, -3) -> (-261.8502, 177.3501, -3)
  line L747 (-261.8502, 177.3501, -3) -> (-261.8502, 180.3501, -3)
  line L748 (-261.8502, 180.3501, -3) -> (-258.8502, 180.3501, -3)
  line L749 (-258.8502, 180.3501, -3) -> (-258.8502, 177.3501, -3)
  line L750 (-258.8502, 177.3501, -3) -> (-255.8502, 177.3501, -3)
  line L751 (-255.8502, 177.3501, -3) -> (-255.8502, 180.3501, -3)
  line L752 (-255.8502, 180.3501, -3) -> (-252.8502, 180.3501, -3)
  line L753 (-252.8502, 180.3501, -3) -> (-252.8502, 177.3501, -3)
  line L754 (-252.8502, 177.3501, -3) -> (-249.8502, 177.3501, -3)
  line L755 (-249.8502, 177.3501, -3) -> (-249.8502, 180.3501, -3)
  line L756 (-249.8502, 180.3501, -3) -> (-246.8502, 180.3501, -3)
  line L757 (-246.8502, 180.3501, -3) -> (-246.8502, 177.3501, -3)
  line L758 (-246.8502, 177.3501, -3) -> (-243.8502, 177.3501, -3)
  line L759 (-243.8502, 177.3501, -3) -> (-243.8502, 180.3501, -3)
  line L760 (-243.8502, 180.3501, -3) -> (-240.8502, 180.3501, -3)
  line L761 (-240.8502, 180.3501, -3) -> (-240.8502, 177.3501, -3)
  line L762 (-240.8502, 177.3501, -3) -> (-237.8502, 177.3501, -3)
  line L763 (-237.8502, 177.3501, -3) -> (-237.8502, 180.3501, -3)
  line L764 (-237.8502, 180.3501, -3) -> (-234.8502, 180.3501, -3)
  line L765 (-234.8502, 180.3501, -3) -> (-234.8502, 177.3501, -3)
  line L766 (-234.8502, 177.3501, -3) -> (-231.8502, 177.3501, -3)
  line L767 (-231.8502, 177.3501, -3) -> (-231.8502, 180.3501, -3)
  line L768 (-231.8502, 180.3501, -3) -> (-228.8502, 180.3501, -3)
  line L769 (-228.8502, 180.3501, -3) -> (-228.8502, 177.3501, -3)
  line L770 (-228.8502, 177.3501, -3) -> (-225.8502, 177.3501, -3)
  line L771 (-225.8502, 177.3501, -3) -> (-225.8502, 180.3501, -3)
  line L772 (-225.8502, 180.3501, -3) -> (-222.8502, 180.3501, -3)
  line L773 (-222.8502, 180.3501, -3) -> (-222.8502, 177.3501, -3)
  line L774 (-222.8502, 177.3501, -3) -> (-219.8502, 177.3501, -3)
  line L775 (-219.8502, 177.3501, -3) -> (-219.8502, 180.3501, -3)
  line L776 (-219.8502, 180.3501, -3) -> (-216.8502, 180.3501, -3)
  line L777 (-216.8502, 180.3501, -3) -> (-216.8502, 177.3501, -3)
  line L778 (-216.8502, 177.3501, -3) -> (-213.8502, 177.3501, -3)
  line L779 (-213.8502, 177.3501, -3) -> (-213.8502, 180.3501, -3)
  line L780 (-213.8502, 180.3501, -3) -> (-210.8502, 180.3501, -3)
  line L781 (-210.8502, 180.3501, -3) -> (-210.8502, 177.3501, -3)
  line L782 (-210.8502, 177.3501, -3) -> (-207.8502, 177.3501, -3)
  line L783 (-207.8502, 177.3501, -3) -> (-207.8502, 180.3501, -3)
  line L784 (-207.8502, 180.3501, -3) -> (-204.8502, 180.3501, -3)
  line L785 (-204.8502, 180.3501, -3) -> (-204.8502, 177.3501, -3)
  line L786 (-204.8502, 177.3501, -3) -> (-201.8502, 177.3501, -3)
  line L787 (-201.8502, 177.3501, -3) -> (-201.8502, 180.3501, -3)
  line L788 (-201.8502, 180.3501, -3) -> (-198.8502, 180.3501, -3)
  line L789 (-198.8502, 180.3501, -3) -> (-198.8502, 177.3501, -3)
  line L790 (-198.8502, 177.3501, -3) -> (-195.8502, 177.3501, -3)
  line L791 (-195.8502, 177.3501, -3) -> (-195.8502, 180.3501, -3)
  line L792 (-195.8502, 180.3501, -3) -> (-192.8502, 180.3501, -3)
  line L793 (-192.8502, 180.3501, -3) -> (-192.8502, 177.3501, -3)
  line L794 (-192.8502, 177.3501, -3) -> (-189.8502, 177.3501, -3)
  line L795 (-189.8502, 177.3501, -3) -> (-189.8502, 180.3501, -3)
  line L796 (-189.8502, 180.3501, -3) -> (-186.8502, 180.3501, -3)
  line L797 (-186.8502, 180.3501, -3) -> (-186.8502, 177.3501, -3)
  line L798 (-186.8502, 177.3501, -3) -> (-183.8502, 177.3501, -3)
  line L799 (-183.8502, 177.3501, -3) -> (-183.8502, 180.3501, -3)
  line L800 (-183.8502, 180.3501, -3) -> (-180.8501, 180.3501, -3)
  line L801 (-180.8501, 180.3501, -3) -> (-180.8501, 177.3501, -3)
  line L802 (-180.8501, 177.3501, -3) -> (-177.8501, 177.3501, -3)
  line L803 (-177.8501, 177.3501, -3) -> (-177.8501, 180.3501, -3)
  line L804 (-177.8501, 180.3501, -3) -> (-174.8501, 180.3501, -3)
  line L805 (-174.8501, 180.3501, -3) -> (-174.8501, 177.3501, -3)
  line L806 (-174.8501, 177.3501, -3) -> (-171.8501, 177.3501, -3)
  line L807 (-171.8501, 177.3501, -3) -> (-171.8501, 180.3501, -3)
  line L808 (-171.8501, 180.3501, -3) -> (-168.8501, 180.3501, -3)
  line L809 (-168.8501, 180.3501, -3) -> (-168.8501, 177.3501, -3)
  line L810 (-168.8501, 177.3501, -3) -> (-165.8501, 177.3501, -3)
  line L811 (-165.8501, 177.3501, -3) -> (-165.8501, 180.3501, -3)
  line L812 (-165.8501, 180.3501, -3) -> (-162.8501, 180.3501, -3)
  line L813 (-162.8501, 180.3501, -3) -> (-162.8501, 177.3501, -3)
  line L814 (-162.8501, 177.3501, -3) -> (-159.8501, 177.3501, -3)
  line L815 (-159.8501, 177.3501, -3) -> (-159.8501, 180.3501, -3)
  line L816 (-159.8501, 180.3501, -3) -> (-156.8501, 180.3501, -3)
  line L817 (-156.8501, 180.3501, -3) -> (-156.8501, 177.3501, -3)
  line L818 (-156.8501, 177.3501, -3) -> (-153.8501, 177.3501, -3)
  line L819 (-153.8501, 177.3501, -3) -> (-153.8501, 180.3501, -3)
  line L820 (-153.8501, 180.3501, -3) -> (-150.8501, 180.3501, -3)
  line L821 (-150.8501, 180.3501, -3) -> (-150.8501, 177.3501, -3)
  line L822 (-150.8501, 177.3501, -3) -> (-147.8501, 177.3501, -3)
  line L823 (-147.8501, 177.3501, -3) -> (-147.8501, 180.3501, -3)
  line L824 (-147.8501, 180.3501, -3) -> (-144.8501, 180.3501, -3)
  line L825 (-144.8501, 180.3501, -3) -> (-144.8501, 177.3501, -3)
  line L826 (-144.8501, 177.3501, -3) -> (-141.8501, 177.3501, -3)
  line L827 (-141.8501, 177.3501, -3) -> (-141.8501, 180.3501, -3)
  line L828 (-141.8501, 180.3501, -3) -> (-138.8501, 180.3501, -3)
  line L829 (-138.8501, 180.3501, -3) -> (-138.8501, 177.3501, -3)
  line L830 (-138.8501, 177.3501, -3) -> (-135.8501, 177.3501, -3)
  line L831 (-135.8501, 177.3501, -3) -> (-135.8501, 180.3501, -3)
  line L832 (-135.8501, 180.3501, -3) -> (-132.8501, 180.3501, -3)
  line L833 (-132.8501, 180.3501, -3) -> (-132.8501, 177.3501, -3)
  line L834 (-132.8501, 177.3501, -3) -> (-129.8501, 177.3501, -3)
  line L835 (-129.8501, 177.3501, -3) -> (-129.8501, 180.3501, -3)
  line L836 (-129.8501, 180.3501, -3) -> (-126.8501, 180.3501, -3)
  line L837 (-126.8501, 180.3501, -3) -> (-126.8501, 177.3501, -3)
  line L838 (-126.8501, 177.3501, -3) -> (-123.8501, 177.3501, -3)
  line L839 (-123.8501, 177.3501, -3) -> (-123.8501, 180.3501, -3)
  line L840 (-123.8501, 180.3501, -3) -> (-120.8501, 180.3501, -3)
  line L841 (-120.8501, 180.3501, -3) -> (-120.8501, 177.3501, -3)
  line L842 (-120.8501, 177.3501, -3) -> (-117.8501, 177.3501, -3)
  line L843 (-117.8501, 177.3501, -3) -> (-117.8501, 180.3501, -3)